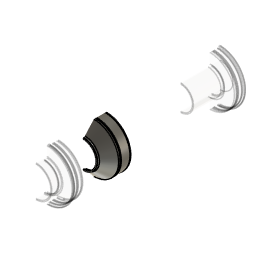
@MK2_EU_Dust_Separator (Autodesk Fusion 360 design; units mm, degrees)
Autodesk Fusion 360 part; units mm, degrees
sketch "Sketch1" plane through (0, 0, 0) normal (1, 0, 0) x (0, 1, 0) in component "MK2_EU_Inlet_Rev_02"
  line L0 (14.5, -71.0875) -> (14.5, -72.1875)
  line L1 (14.5, -72.1875) -> (28, -72.1875)
  line L2 (-5, -73.6875) -> (-3, -75.6875)
  line L3 (0, -75.6875) -> (0, -71.1875)
  line L4 (3.5, -71.1875) -> (3.5, -72.1875)
  line L5 (-7.812, -40.5) -> (-13.5, -40.5)
  line L6 (28, -72.1875) -> (28, -69.5)
  arc A0 (14.5, -71.0875) -> (11, -71.0875) centre (12.75, -71.0875) ccw
  line L7 (-37, -46.5) -> (-5, -46.5)
  line L8 (28, -69.5) -> (-7.812, -40.5)
  arc A1 (3.5, -71.1875) -> (0, -71.1875) centre (1.75, -71.1875) ccw
  line L9 (11, -72.1875) -> (11, -71.0875)
  line L10 (-13.5, -40.5) -> (-13.5, -43.5)
  line L11 (-5, -46.5) -> (-5, -73.6875)
  line L12 (3.5, -72.1875) -> (11, -72.1875)
  line L13 (-13.5, -43.5) -> (-37, -43.5)
  line L14 (-37, 0) -> (28, 0)
  line L15 (-37, -43.5) -> (-37, -46.5)
  line L16 (-3, -75.6875) -> (0, -75.6875)
  dimension "d19" = 65
  dimension "d20" = 3
  dimension "d21" = 81
  dimension "d22" = 3
  dimension "d23" = 23.5
  dimension "d24" = 39
  dimension "d25" = 3.5
  dimension "d26" = 5
  dimension "d27" = 135
  dimension "d28" = 3
  dimension "d29" = 32
  dimension "d30" = 3.5
  dimension "d31" = 1
  dimension "d32" = 1.1
  dimension "d33" = 28
  dimension "d34" = 11
  dimension "d35" = 144.375
  dimension "d36" = 139
  constraint horizontal L14
  constraint parallel L7 L14
  constraint perpendicular L11 L14
  constraint perpendicular L11 L16
  constraint perpendicular L3 L14
  constraint tangent L3 A1
  constraint tangent L4 A1
  constraint parallel L3 L4
  constraint perpendicular L4 L12
  constraint perpendicular L9 L12
  constraint tangent A0 L9
  constraint tangent L0 A0
  constraint parallel L0 L9
  constraint perpendicular L0 L1
  constraint perpendicular L1 L6
  constraint perpendicular L5 L6
  constraint perpendicular L5 L10
  constraint perpendicular L10 L13
  constraint perpendicular L7 L15
  constraint equal A0 A1
  constraint collinear L1 L12
  constraint coincident L14.start L15
  constraint coincident origin L14
  constraint coincident L3 origin
  constraint coincident L14 origin
  measures "d19" distance of L14.end L14.start
  measures "d20" distance of L7 L13
  measures "d22" distance of L5 L13
  measures "d23" distance of L10 L15
  measures "d24" angle of L8 L14
  measures "d25" distance of L12 L16
  measures "d26" distance of L3 L11
  measures "d27" angle of L2 L16
  measures "d28" distance of L3.start L2.end
  measures "d29" distance of L11 L15
  measures "d30" diameter of A1
  measures "d31" distance of A1.centre L12
  measures "d32" distance of A0.centre L12
  measures "d33" distance of L3.start L6
  measures "d34" horizontal distance of A0.centre A1.centre
revolve "Revolve1" add sketch "Sketch1" angle 360 about axis through (0, 0, 0) along (0, 1, 0) makes body 1 in component "MK2_EU_Inlet_Rev_02"
sketch "Sketch2" plane through (0, 28, 0) normal (0, 1, 0) x (-1, 0, 0) in component "MK2_EU_Inlet_Rev_02"
  circle A0 centre (0, 0) radius 69.5
  circle A1 centre (0, 0) radius 72.1875
  line L0 (0, 0) -> (-19.2913, -69.5621)
  line L1 (0, 0) -> (19.2913, -69.5621)
  arc A2 (-19.2913, -69.5621) -> (19.2913, -69.5621) centre (0, 0) ccw
  line L2 (0, 0) -> (0, -72.1875) construction
  dimension "d40" = 31
  constraint coincident A0.centre A1.centre
  constraint coincident A1 L0.end
  constraint coincident A1 L1.end
  constraint midpoint A2 L2.end
  constraint vertical L2
  measures "d40" angle of L0 L1
extrude "Extrude1" cut sketch "Sketch2" against normal blind 3 contours A0 L0 L1 | A0 A1 L0 L1 A2 picked at (9.3151, -45.2792) bodies 1 in component "MK2_EU_Inlet_Rev_02"
fillet "Fillet1" radius 10 1 edges at (-37.7593, -7.812, -14.6454) on bodies 1 in component "MK2_EU_Inlet_Rev_02"
chamfer "Chamfer1" distance 5 distance2 0.5 1 edges at (0, 28, 72.1875) measured on face at (-5.3662, 19, 71.9878) on bodies 1 in component "MK2_EU_Inlet_Rev_02"
sketch "Sketch1 (2)" plane through (0, 0, 0) normal (1, 0, 0) x (0, 1, 0) in component "MK2_EU_Outlet_Rev_02"
  line L0 (0, 0) -> (500, 0)
  line L1 (495, -75.6875) -> (495, -71.1875)
  arc A0 (495, -71.1875) -> (491.5, -71.1875) centre (493.25, -71.1875) ccw
  line L2 (491.5, -71.1875) -> (491.5, -72.1875)
  line L3 (491.5, -72.1875) -> (481.75, -72.1875)
  line L4 (481.75, -72.1875) -> (481.75, -71.0875)
  arc A1 (481.75, -71.0875) -> (478.25, -71.0875) centre (480, -71.0875) ccw
  line L5 (478.25, -71.0875) -> (478.25, -72.1875)
  line L6 (478.25, -72.1875) -> (470, -72.1875)
  line L7 (470, -72.1875) -> (470, -37.5)
  line L8 (470, -37.5) -> (383.375, -37.5)
  line L9 (383.375, -37.5) -> (383.375, -34.5)
  line L10 (383.375, -34.5) -> (475, -34.5)
  line L11 (475, -34.5) -> (475, -37.5)
  line L12 (475, -37.5) -> (500, -37.5)
  line L13 (500, -37.5) -> (500, -73.6875)
  line L14 (500, -73.6875) -> (498, -75.6875)
  line L15 (498, -75.6875) -> (495, -75.6875)
  dimension "d45" = 3
  dimension "d47" = 3.5
  dimension "d48" = 1
  dimension "d49" = 1.1
  dimension "d50" = 10
  dimension "d51" = 25
  dimension "d52" = 5
  dimension "d53" = 144.375
  dimension "d54" = 3
  dimension "d55" = 45
  dimension "d56" = 25
  dimension "d57" = 3.5
  dimension "d58" = 86.625
  dimension "d59" = 495
  dimension "d69" = 75
  dimension "d70" = 69
  constraint coincident L0.start origin
  constraint horizontal L0
  constraint perpendicular L0 L1
  constraint tangent L1 A0
  constraint tangent A0 L2
  constraint perpendicular L0 L2
  constraint perpendicular L2 L3
  constraint perpendicular L3 L4
  constraint tangent L4 A1
  constraint tangent A1 L5
  constraint perpendicular L3 L5
  constraint perpendicular L5 L6
  constraint perpendicular L6 L7
  constraint perpendicular L5 L8
  constraint perpendicular L8 L9
  constraint perpendicular L9 L10
  constraint perpendicular L10 L11
  constraint perpendicular L11 L12
  constraint perpendicular L12 L13
  constraint perpendicular L13 L15
  constraint coincident L1.start L15.end
  constraint equal A0 A1
  constraint collinear L3 L6
  constraint coincident L0.end L13
  measures "d45" distance of L8.end L9.end
  measures "d47" diameter of A0
  measures "d48" distance of A0.centre L3
  measures "d49" distance of L3 A1.centre
  measures "d50" distance of A1.centre L7
  measures "d51" distance of L1 L7
  measures "d52" distance of L1 L13
  measures "d54" distance of L1 L14.end
  measures "d55" angle of L14 L15
  measures "d56" distance of L11 L13
  measures "d57" distance of L3 L15
  measures "d58" distance of L7 L9
  measures "d59" distance of L0.start L1
revolve "Revolve1'" add sketch "Sketch1 (2)" angle 360 about axis through (0, 0, 0) along (0, 1, 0) separate body makes body 2 in component "MK2_EU_Outlet_Rev_02"
chamfer "Chamfer1'" distance 0.5 distance2 5 1 edges at (-67.3024, 470, -26.1041) measured on face at (5.4494, 470, -60.2166) on bodies 2 in component "MK2_EU_Outlet_Rev_02"
fillet "Fillet1'" radius 5 1 edges at (-34.9623, 470, -13.5606) on bodies 2 in component "MK2_EU_Outlet_Rev_02"
fillet "Fillet1'" radius 1.5 1 edges at (-34.9623, 383.375, -13.5606) on bodies 2 in component "MK2_EU_Outlet_Rev_02"
fillet "Fillet2" radius 1.5 1 edges at (-32.1653, 383.375, -12.4757) on bodies 2 in component "MK2_EU_Outlet_Rev_02"
sketch "Sketch1 (3)" plane through (0, 0, 0) normal (1, 0, 0) x (0, 1, 0) in component "MK2_EU_Impeller_Shroud"
  line L0 (0, 0) -> (168.068, 0)
  line L1 (168.068, 69.5) -> (143.068, 69.5)
  line L2 (143.068, 69.5) -> (105.5278, 38)
  line L3 (105.5278, 38) -> (100.5278, 38)
  arc A0 (100.5278, 41) -> (100.5278, 38) centre (100.5278, 39.5) ccw
  line L4 (100.5278, 41) -> (104.1805, 41)
  line L5 (104.1805, 41) -> (131.9, 72.185)
  line L6 (131.9, 72.185) -> (136.318, 72.185)
  line L7 (136.318, 72.185) -> (136.318, 70.935)
  arc A1 (136.318, 70.935) -> (139.818, 70.935) centre (138.068, 70.935) ccw
  line L8 (139.818, 70.935) -> (139.818, 72.185)
  line L9 (139.818, 72.185) -> (165.068, 72.185)
  line L10 (165.068, 72.185) -> (168.068, 71.585)
  line L11 (168.068, 71.585) -> (168.068, 69.5)
  dimension "d71" = 168.068
  dimension "d72" = 1.25
  dimension "d73" = 0.6
  dimension "d74" = 3
  dimension "d75" = 30
  dimension "d76" = 3.5
  dimension "d77" = 144.37
  dimension "d78" = 139
  dimension "d79" = 82
  dimension "d80" = 5
  dimension "d81" = 3
  dimension "d82" = 40
  dimension "d83" = 36.168
  dimension "d84" = 25
  dimension "d85" = 3
  constraint coincident L0.start origin
  constraint horizontal L0
  constraint horizontal L1
  constraint parallel L1 L3
  constraint tangent L3 A0
  constraint tangent A0 L4
  constraint parallel L3 L4
  constraint parallel L4 L6
  constraint perpendicular L6 L7
  constraint tangent L7 A1
  constraint tangent A1 L8
  constraint parallel L7 L8
  constraint perpendicular L7 L9
  constraint vertical L11
  constraint coincident L0.end L11
  constraint collinear L6 L9
  measures "d71" distance of L0.start L0.end
  measures "d72" distance of L6.end L7.end
  measures "d73" distance of L9 L10.end
  measures "d74" distance of L9.end L11
  measures "d75" distance of A1.centre L11
  measures "d76" diameter of A1
  measures "d80" horizontal distance of L2.end A0.centre
  measures "d81" distance of L2.end L5
  measures "d82" angle of L0 L2
  measures "d83" distance of L5.end L11
  measures "d84" distance of L1.start L1.end
  measures "d85" distance of L3 L4
revolve "Revolve1''" add sketch "Sketch1 (3)" angle 360 about axis through (0, 0, 0) along (0, 1, 0) separate body makes body 3 in component "MK2_EU_Impeller_Shroud"
ref_plane "WorkPlane1" through (0, 135.1, 0) normal (0, 1, 0) x (0, 0, 1) in component "MK2_EU_Impeller_Shroud"
sketch "Sketch2 (2)" plane through (0, 135.1, 0) normal (0, 1, 0) x (1, 0, 0) in component "MK2_EU_Impeller_Shroud"
  line L0 (0, 0) -> (-19.2906, 69.5597)
  line L1 (19.2906, 69.5597) -> (0, 0)
  line L2 (0, 0) -> (0, 81.8921) construction
  arc A0 (19.2906, 69.5597) -> (-19.2906, 69.5597) centre (0, 0) ccw
  circle A1 centre (0, 0) radius 72.185
  arc A2 (17.1527, 61.8506) -> (-17.1527, 61.8506) centre (0, 0) ccw
  dimension "d88" = 31
  dimension "d89" = -8
  constraint coincident L0.start L1.end
  constraint vertical L2
  constraint coincident L1 A0.start
  constraint coincident L0 A0.end
  constraint coincident L1.start A0.start
  constraint coincident L0.end A0.end
  constraint equal A0 A1
  measures "d88" angle of L0 L1
extrude "Extrude1'" cut sketch "Sketch2 (2)" along normal blind 0.5 and the other way blind 3.1 contours L0 L1 A0 A1 A2 bodies 3 in component "MK2_EU_Impeller_Shroud"
fillet "Fillet1''" radius 5 1 edges at (-38.2254, 104.1805, 14.8262) on bodies 3 in component "MK2_EU_Impeller_Shroud"
fillet "Fillet1''" radius 10 1 edges at (-35.4284, 105.5278, 13.7414) on bodies 3 in component "MK2_EU_Impeller_Shroud"
component "MK2_EU_Inlet_Rev_02" placed x (1, 0, 0) y (0, 1, 0) z (0, 0, 1) at (0, 0, 0)
component "MK2_EU_Outlet_Rev_02" placed x (1, 0, 0) y (0, 1, 0) z (0, 0, 1) at (0, 0, 0)
component "MK2_EU_Impeller_Shroud" placed x (1, 0, 0) y (0, 1, 0) z (0, 0, 1) at (0, 0, 0)
equation "d58 = d53 * 0.6"
